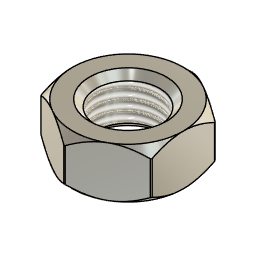
assignment1c-hexnut (Autodesk Fusion 360 design; units mm, degrees)
Autodesk Fusion 360 part; units mm, degrees
sketch "Sketch1" plane through (0, 0, 0) normal (0, 0, 1) x (1, 0, 0) in component "Hex nut"
  line L0 (8.3, 4.792) -> (0, 9.584)
  line L1 (0, 9.584) -> (-8.3, 4.792)
  line L2 (-8.3, 4.792) -> (-8.3, -4.792)
  line L3 (-8.3, -4.792) -> (0, -9.584)
  line L4 (0, -9.584) -> (8.3, -4.792)
  line L5 (8.3, -4.792) -> (8.3, 4.792)
  dimension "d5" = 16.6
  constraint vertical L2
  measures "d5" distance of L2 L5
extrude "Extrude1" add sketch "Sketch1" along normal blind 7.5 in component "Hex nut"
sketch "Sketch2" plane through (0, 0, 7.5) normal (0, 0, 1) x (-1, 0, 0) in component "Hex nut"
  line L0 (-8.3, 4.792) -> (-8.3, -4.792)
  line L1 (-8.3, -4.792) -> (0, -9.584)
  line L2 (0, -9.584) -> (8.3, -4.792)
  line L3 (8.3, -4.792) -> (8.3, 4.792)
  line L4 (8.3, 4.792) -> (0, 9.584)
  line L5 (0, 9.584) -> (-8.3, 4.792)
  circle A0 centre (0, 0) radius 8.3
  constraint coincident A0.centre origin
  constraint tangent L1 A0
extrude "Extrude2" cut sketch "Sketch2" against normal blind 7.5 draft 45 contours A0 keep common part in component "Hex nut"
ref_plane "WorkPlane1" through (0, 0, 3.75) normal (0, 0, 1) x (1, 0, 0) in component "Hex nut"
mirror "Mirror1" about plane through (0, 0, 3.75) normal (0, 0, 1) of "Extrude2" in component "Hex nut"
hole "Hole1" at (0, 0, 7.5) direction (0, 0, -1) diameter 8.7 end through all in component "Hex nut"
thread "Thread1" "ISO Metric profile 11.0 M11x1.5 6H" major diameter 11.1933 minor diameter 9.5262 pitch 1.5 angle 60 resizes the face on face at (0.4331, -4.3284, 5) from (0, 0, 7.2) to (0, 0, 0.7) in component "Hex nut"
chamfer "Chamfer1" distance 1 angle 45 2 edges at (-4.4408, 1.7224, 7.5) (-4.4408, -1.7224, 0) in component "Hex nut"
fillet "Fillet1" radius 0.2 5 edges at (8.3, -4.792, 3.75) (0, -9.584, 3.75) (8.3, 4.792, 3.75) (0, 9.584, 3.75) (-8.3, 4.792, 3.75) in component "Hex nut"
fillet "Fillet2" radius 0.2 1 edges at (-8.3, -4.792, 3.75) in component "Hex nut"
component "Hex nut" placed x (1, 0, 0) y (0, 1, 0) z (0, 0, 1) at (0, 0, 0)
